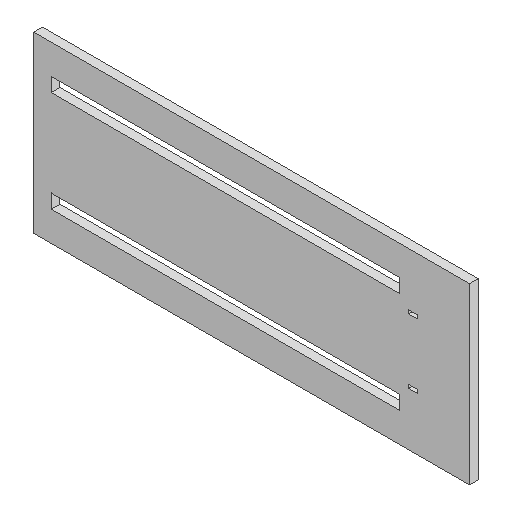
# Autodesk Inventor part: Team29_BoxLid
Saved by Autodesk Inventor 2023 (Build 270158000, 158)
## iProperties
Created: 2023-02-27
Part Number: Team29_BoxLid
Material: Generic
Document SubType Name: Modeling
Designer: Fariha
Density: 1 g/cm^3
Appearance: Default
Author: Fariha
Autodesk Inventor part; units mm, degrees
ref_plane "YZ Plane" through (0, 0, 0) normal (1, 0, 0) x (0, 1, 0)
ref_plane "XZ Plane" through (0, 0, 0) normal (0, 1, 0) x (-1, 0, 0)
ref_plane "XY Plane" through (0, 0, 0) normal (0, 0, 1) x (1, 0, 0)
sketch "Sketch1" plane through (0, 0, 0) normal (0, 0, 1) x (1, 0, 0)
  line L0 (-125, 60) -> (125, 60)
  line L1 (125, 60) -> (125, -40)
  line L2 (125, -40) -> (-125, -40)
  line L3 (-125, -40) -> (-125, 60)
  line L4 (-115, -15) -> (85, -15)
  line L5 (85, -15) -> (85, -23)
  line L6 (85, -23) -> (-115, -23)
  line L7 (-115, -23) -> (-115, -15)
  line L8 (-115, 43) -> (85, 43)
  line L9 (85, 43) -> (85, 35)
  line L10 (85, 35) -> (-115, 35)
  line L11 (-115, 35) -> (-115, 43)
  line L12 (90, 29.5) -> (95, 29.5)
  line L13 (95, 29.5) -> (95, 27.5)
  line L14 (95, 27.5) -> (90, 27.5)
  line L15 (90, 27.5) -> (90, 29.5)
  line L16 (90, -7.5) -> (95, -7.5)
  line L17 (95, -7.5) -> (95, -9.5)
  line L18 (95, -9.5) -> (90, -9.5)
  line L19 (90, -9.5) -> (90, -7.5)
  point P0 (0, 0)
  point P1 (-115, 39)
  point P2 (92.5, -7.5)
  point P3 (92.5, 27.5)
  point P4 (92.5, -9.5)
  point P5 (95, 28.5)
  dimension "d0" = 250
  dimension "d1" = 100
  dimension "d2" = 125
  dimension "d3" = 60
  dimension "d4" = 200
  dimension "d5" = 8
  dimension "d6" = 8
  dimension "d7" = 50
  dimension "d8" = 17
  dimension "d9" = 10
  dimension "d10" = 5
  dimension "d11" = 2
  dimension "d12" = 2
  dimension "d13" = 35
  dimension "d14" = 30.5
  dimension "d15" = 30
  constraints: 40 end point, 10 parallel, 5 horizontal, 5 midpoint, 5 perpendicular, 4 point on line
  measures "d0" distance of L1.end L2.end
  measures "d1" distance of L0.end L1.end
  measures "d2" distance from line of point (0, 0) L3
  measures "d3" distance from line of L0 point (0, 0)
  measures "d4" distance of L5.end L6.end
  measures "d5" distance of L4.end L5.end
  measures "d6" distance of L8.end L9.end
  measures "d7" distance between parallel lines of L4 L10
  measures "d8" distance between parallel lines of L0 L8
  measures "d9" distance from line of L3 point (-115, 39)
  measures "d10" distance of L13.end L14.end
  measures "d11" distance of L12.end L13.end
  measures "d12" distance of L16.end L17.end
  measures "d13" distance of point (92.5, -7.5) point (92.5, 27.5)
  measures "d14" distance from line of L2 point (92.5, -9.5)
  measures "d15" distance from line of L1 point (95, 28.5)
extrude "Extrusion1" add sketch "Sketch1" along normal blind 5
body "Solid1"
